Autodesk Inventor part; units mm, degrees
(part 2 of 2)
  arc A229 (57.1329, 113.815) -> (59.0329, 111.915) centre (59.0329, 113.815) ccw
  line L194 (78.8671, 123.4514) -> (78.8671, 113.815)
  arc A230 (78.8671, 123.4514) -> (76.9671, 125.3514) centre (76.9671, 123.4514) ccw
  line L195 (76.9671, 125.3514) -> (71.42, 125.3514)
  line L196 (71.42, 111.915) -> (76.9671, 111.915)
  arc A231 (76.9671, 111.915) -> (78.8671, 113.815) centre (76.9671, 113.815) ccw
  arc A232 (64.58, 125.3514) -> (71.42, 125.3514) centre (68, 128.8174) ccw
  arc A233 (71.42, 111.915) -> (64.58, 111.915) centre (68, 108.495) ccw
  line L197 (57.1329, 12.5486) -> (57.1329, 22.185)
  arc A234 (57.1329, 12.5486) -> (59.0329, 10.6486) centre (59.0329, 12.5486) ccw
  line L198 (59.0329, 10.6486) -> (64.58, 10.6486)
  line L199 (64.58, 24.085) -> (59.0329, 24.085)
  arc A235 (59.0329, 24.085) -> (57.1329, 22.185) centre (59.0329, 22.185) ccw
  line L200 (78.8671, 12.5486) -> (78.8671, 22.185)
  arc A236 (76.9671, 10.6486) -> (78.8671, 12.5486) centre (76.9671, 12.5486) ccw
  line L201 (76.9671, 10.6486) -> (71.42, 10.6486)
  line L202 (71.42, 24.085) -> (76.9671, 24.085)
  arc A237 (78.8671, 22.185) -> (76.9671, 24.085) centre (76.9671, 22.185) ccw
  arc A238 (71.42, 10.6486) -> (64.58, 10.6486) centre (68, 7.1826) ccw
  arc A239 (64.58, 24.085) -> (71.42, 24.085) centre (68, 27.505) ccw
  arc A240 (27.6448, 91.2527) -> (44.7476, 108.3555) centre (-2.445, 138.4453) ccw
  arc A241 (27.6448, 91.2527) -> (28.102, 89.6852) centre (28.102, 90.5356) ccw
  arc A242 (46.3151, 107.8983) -> (44.7476, 108.3555) centre (45.4647, 107.8983) ccw
  line L203 (40.2804, 87.1341) -> (22.5335, 87.1334)
  line L204 (44.1891, 89.6852) -> (28.102, 89.6852)
  line L205 (46.3151, 91.8112) -> (46.3151, 107.8983)
  arc A243 (44.1891, 89.6852) -> (46.3151, 91.8112) centre (44.1891, 91.8112) ccw
  arc A244 (27.1963, 78.4533) -> (28.6868, 78.3895) centre (28.007, 79.9485) ccw
  arc A245 (28.6868, 78.3895) -> (40.8045, 85.614) centre (6.3199, 129.6804) ccw
  line L206 (21.3459, 81.6253) -> (27.1963, 78.4533)
  line L207 (30.5408, 76.64) -> (37.2048, 73.0269)
  arc A246 (40.8045, 85.614) -> (40.2804, 87.1341) centre (40.2804, 86.2837) ccw
  arc A247 (91.2524, 108.3555) -> (108.3552, 91.2527) centre (138.445, 138.4453) ccw
  arc A248 (107.898, 89.6852) -> (108.3552, 91.2527) centre (107.898, 90.5356) ccw
  arc A249 (91.2524, 108.3555) -> (89.6849, 107.8983) centre (90.5353, 107.8983) ccw
  line L208 (91.8109, 89.6852) -> (107.898, 89.6852)
  line L209 (89.6849, 91.8112) -> (89.6849, 107.8983)
  arc A250 (89.6849, 91.8112) -> (91.8109, 89.6852) centre (91.8109, 91.8112) ccw
  arc A251 (108.3552, 44.7479) -> (91.2524, 27.6451) centre (138.445, -2.4447) ccw
  arc A252 (108.3552, 44.7479) -> (107.898, 46.3154) centre (107.898, 45.465) ccw
  arc A253 (89.6849, 28.1023) -> (91.2524, 27.6451) centre (90.5353, 28.1023) ccw
  line L210 (91.8109, 46.3154) -> (107.898, 46.3154)
  line L211 (89.6849, 44.1894) -> (89.6849, 28.1023)
  arc A254 (91.8109, 46.3154) -> (89.6849, 44.1894) centre (91.8109, 44.1894) ccw
  arc A255 (30.5752, 77.4043) -> (44.1261, 85.6969) centre (8.4389, 128.7951) ccw
  arc A256 (44.7901, 85.2067) -> (44.1261, 85.6969) centre (44.3973, 85.3694) ccw
  arc A257 (30.5752, 77.4043) -> (30.5408, 76.64) centre (30.7434, 77.0138) ccw
  line L212 (44.7901, 85.2067) -> (40.1822, 74.0823)
  arc A258 (37.2048, 73.0269) -> (40.1822, 74.0823) centre (38.2181, 74.8959) ccw
  line L213 (30.5408, 59.3606) -> (37.2048, 62.9737)
  arc A259 (40.1822, 61.9183) -> (37.2048, 62.9737) centre (38.2181, 61.1047) ccw
  arc A260 (44.1261, 50.3037) -> (30.5752, 58.5963) centre (8.4389, 7.2055) ccw
  arc A261 (44.1261, 50.3037) -> (44.7901, 50.7939) centre (44.3973, 50.6312) ccw
  arc A262 (30.5408, 59.3606) -> (30.5752, 58.5963) centre (30.7434, 58.9868) ccw
  line L214 (44.7901, 50.7939) -> (40.1822, 61.9183)
  line L215 (105.4592, 76.64) -> (98.7952, 73.0269)
  arc A263 (91.8739, 85.6969) -> (105.4248, 77.4043) centre (127.5611, 128.7951) ccw
  arc A264 (91.8739, 85.6969) -> (91.2099, 85.2067) centre (91.6027, 85.3694) ccw
  arc A265 (105.4592, 76.64) -> (105.4248, 77.4043) centre (105.2566, 77.0138) ccw
  line L216 (91.2099, 85.2067) -> (95.8178, 74.0823)
  arc A266 (95.8178, 74.0823) -> (98.7952, 73.0269) centre (97.7819, 74.8959) ccw
  line L217 (105.4592, 59.3606) -> (98.7952, 62.9737)
  arc A267 (98.7952, 62.9737) -> (95.8178, 61.9183) centre (97.7819, 61.1047) ccw
  arc A268 (105.4248, 58.5963) -> (91.8739, 50.3037) centre (127.5611, 7.2055) ccw
  arc A269 (91.2099, 50.7939) -> (91.8739, 50.3037) centre (91.6027, 50.6312) ccw
  arc A270 (105.4248, 58.5963) -> (105.4592, 59.3606) centre (105.2566, 58.9868) ccw
  line L218 (91.2099, 50.7939) -> (95.8178, 61.9183)
  line L219 (59.3603, 105.4595) -> (62.9734, 98.7955)
  arc A271 (61.918, 95.8181) -> (62.9734, 98.7955) centre (61.1044, 97.7822) ccw
  arc A272 (50.3034, 91.8742) -> (58.596, 105.4251) centre (7.2052, 127.5614) ccw
  arc A273 (50.3034, 91.8742) -> (50.7936, 91.2102) centre (50.6309, 91.603) ccw
  arc A274 (59.3603, 105.4595) -> (58.596, 105.4251) centre (58.9865, 105.2569) ccw
  line L220 (50.7936, 91.2102) -> (61.918, 95.8181)
  line L221 (76.6397, 105.4595) -> (73.0266, 98.7955)
  arc A275 (73.0266, 98.7955) -> (74.082, 95.8181) centre (74.8956, 97.7822) ccw
  arc A276 (77.404, 105.4251) -> (85.6966, 91.8742) centre (128.7948, 127.5614) ccw
  arc A277 (85.2064, 91.2102) -> (85.6966, 91.8742) centre (85.3691, 91.603) ccw
  arc A278 (77.404, 105.4251) -> (76.6397, 105.4595) centre (77.0135, 105.2569) ccw
  line L222 (85.2064, 91.2102) -> (74.082, 95.8181)
  line L223 (59.3603, 30.5411) -> (62.9734, 37.2051)
  arc A279 (62.9734, 37.2051) -> (61.918, 40.1825) centre (61.1044, 38.2184) ccw
  arc A280 (58.596, 30.5755) -> (50.3034, 44.1264) centre (7.2052, 8.4392) ccw
  arc A281 (50.7936, 44.7904) -> (50.3034, 44.1264) centre (50.6309, 44.3976) ccw
  arc A282 (58.596, 30.5755) -> (59.3603, 30.5411) centre (58.9865, 30.7437) ccw
  line L224 (50.7936, 44.7904) -> (61.918, 40.1825)
  line L225 (76.6397, 30.5411) -> (73.0266, 37.2051)
  arc A283 (85.6966, 44.1264) -> (77.404, 30.5755) centre (128.7948, 8.4392) ccw
  arc A284 (85.6966, 44.1264) -> (85.2064, 44.7904) centre (85.3691, 44.3976) ccw
  arc A285 (76.6397, 30.5411) -> (77.404, 30.5755) centre (77.0135, 30.7437) ccw
  line L226 (85.2064, 44.7904) -> (74.082, 40.1825)
  arc A286 (74.082, 40.1825) -> (73.0266, 37.2051) centre (74.8956, 38.2184) ccw
  circle A287 centre (68, 68) radius 24.5933
  arc A288 (44.7476, 27.6451) -> (27.6448, 44.7479) centre (-2.445, -2.4447) ccw
  arc A289 (44.7476, 27.6451) -> (46.3151, 28.1023) centre (45.4647, 28.1023) ccw
  arc A290 (28.102, 46.3154) -> (27.6448, 44.7479) centre (28.102, 45.465) ccw
  line L227 (46.3151, 44.1894) -> (46.3151, 28.1023)
  line L228 (44.1891, 46.3154) -> (28.102, 46.3154)
  arc A291 (46.3151, 44.1894) -> (44.1891, 46.3154) centre (44.1891, 44.1894) ccw
  line L229 (64.2924, 102.9057) -> (67.1209, 97.6888)
  arc A292 (67.1209, 97.6888) -> (68.8791, 97.6888) centre (68, 98.1654) ccw
  line L230 (71.7076, 102.9057) -> (68.8791, 97.6888)
  arc A293 (65.6558, 104.2572) -> (70.3442, 104.2572) centre (68, 108.4916) ccw
  arc A294 (65.6558, 104.2572) -> (64.2924, 102.9057) centre (65.1715, 103.3823) ccw
  arc A295 (71.7076, 102.9057) -> (70.3442, 104.2572) centre (70.8285, 103.3823) ccw
  line L231 (64.2924, 33.0943) -> (67.1209, 38.3112)
  arc A296 (68.8791, 38.3112) -> (67.1209, 38.3112) centre (68, 37.8346) ccw
  line L232 (71.7076, 33.0943) -> (68.8791, 38.3112)
  arc A297 (70.3442, 31.7428) -> (65.6558, 31.7428) centre (68, 27.5084) ccw
  arc A298 (64.2924, 33.0943) -> (65.6558, 31.7428) centre (65.1715, 32.6177) ccw
  arc A299 (70.3442, 31.7428) -> (71.7076, 33.0943) centre (70.8285, 32.6177) ccw
  line L233 (33.0946, 71.7079) -> (38.3115, 68.8794)
  arc A300 (38.3115, 67.1212) -> (38.3115, 68.8794) centre (37.8349, 68.0003) ccw
  line L234 (33.0946, 64.2927) -> (38.3115, 67.1212)
  arc A301 (31.7431, 65.6561) -> (31.7431, 70.3445) centre (27.5087, 68.0003) ccw
  arc A302 (33.0946, 71.7079) -> (31.7431, 70.3445) centre (32.618, 70.8288) ccw
  arc A303 (31.7431, 65.6561) -> (33.0946, 64.2927) centre (32.618, 65.1718) ccw
  line L235 (102.906, 71.7079) -> (97.6891, 68.8794)
  arc A304 (97.6891, 68.8794) -> (97.6891, 67.1212) centre (98.1657, 68.0003) ccw
  line L236 (102.906, 64.2927) -> (97.6891, 67.1212)
  arc A305 (104.2575, 70.3445) -> (104.2575, 65.6561) centre (108.4919, 68.0003) ccw
  arc A306 (104.2575, 70.3445) -> (102.906, 71.7079) centre (103.3826, 70.8288) ccw
  arc A307 (102.906, 64.2927) -> (104.2575, 65.6561) centre (103.3826, 65.1718) ccw
  circle A308 centre (7.7484, 68) radius 1.6
  circle A309 centre (128.2516, 68) radius 1.6
  circle A310 centre (68, 128.2516) radius 1.6
  circle A311 centre (68, 7.7484) radius 1.6
  arc A312 (4.7048, 71.2684) -> (4.7048, 64.7316) centre (8.3141, 68) ccw
  arc A313 (5.9986, 61.3754) -> (4.7048, 64.7316) centre (0.9986, 61.3754) ccw
  arc A314 (4.7048, 71.2684) -> (5.9986, 74.6246) centre (0.9986, 74.6246) ccw
  arc A315 (131.2952, 64.7316) -> (131.2952, 71.2684) centre (127.6859, 68) ccw
  arc A316 (131.2952, 64.7316) -> (130.0014, 61.3754) centre (135.0014, 61.3754) ccw
  arc A317 (130.0014, 74.6246) -> (131.2952, 71.2684) centre (135.0014, 74.6246) ccw
  arc A318 (71.2684, 131.2952) -> (64.7316, 131.2952) centre (68, 127.6859) ccw
  arc A319 (71.2684, 131.2952) -> (74.6246, 130.0014) centre (74.6246, 135.0014) ccw
  arc A320 (61.3754, 130.0014) -> (64.7316, 131.2952) centre (61.3754, 135.0014) ccw
  arc A321 (64.7316, 4.7048) -> (71.2684, 4.7048) centre (68, 8.3141) ccw
  arc A322 (64.7316, 4.7048) -> (61.3754, 5.9986) centre (61.3754, 0.9986) ccw
  arc A323 (74.6246, 5.9986) -> (71.2684, 4.7048) centre (74.6246, 0.9986) ccw
  line L237 (17, 83.6623) -> (17, 82.8671)
  arc A324 (18.2965, 85.5345) -> (21.7007, 86.9517) centre (-0.1983, 134.7566) ccw
  arc A325 (18.2965, 85.5345) -> (17, 83.6623) centre (19, 83.6623) ccw
  arc A326 (22.5335, 87.1334) -> (21.7007, 86.9517) centre (22.5336, 85.1334) ccw
  line L238 (18, 81.8671) -> (20.3926, 81.8671)
  arc A327 (17, 82.8671) -> (18, 81.8671) centre (18, 82.8671) ccw
  arc A328 (21.3459, 81.6253) -> (20.3926, 81.8671) centre (20.3926, 79.8671) ccw
  line L239 (40.2804, 48.8659) -> (22.5335, 48.8666)
  arc A329 (28.6868, 57.6105) -> (27.1963, 57.5467) centre (28.007, 56.0515) ccw
  arc A330 (40.8045, 50.386) -> (28.6868, 57.6105) centre (6.3199, 6.3196) ccw
  line L240 (21.3459, 54.3747) -> (27.1963, 57.5467)
  arc A331 (40.2804, 48.8659) -> (40.8045, 50.386) centre (40.2804, 49.7163) ccw
  line L241 (17, 52.3377) -> (17, 53.1329)
  arc A332 (21.7007, 49.0483) -> (18.2965, 50.4655) centre (-0.1983, 1.2434) ccw
  arc A333 (17, 52.3377) -> (18.2965, 50.4655) centre (19, 52.3377) ccw
  arc A334 (21.7007, 49.0483) -> (22.5335, 48.8666) centre (22.5336, 50.8666) ccw
  line L242 (18, 54.1329) -> (20.3926, 54.1329)
  arc A335 (18, 54.1329) -> (17, 53.1329) centre (18, 53.1329) ccw
  arc A336 (20.3926, 54.1329) -> (21.3459, 54.3747) centre (20.3926, 56.1329) ccw
  line L243 (95.7196, 87.1341) -> (113.4665, 87.1334)
  arc A337 (107.3132, 78.3895) -> (108.8037, 78.4533) centre (107.993, 79.9485) ccw
  arc A338 (95.1955, 85.614) -> (107.3132, 78.3895) centre (129.6801, 129.6804) ccw
  line L244 (114.6541, 81.6253) -> (108.8037, 78.4533)
  arc A339 (95.7196, 87.1341) -> (95.1955, 85.614) centre (95.7196, 86.2837) ccw
  line L245 (119, 83.6623) -> (119, 82.8671)
  arc A340 (114.2993, 86.9517) -> (117.7035, 85.5345) centre (136.1983, 134.7566) ccw
  arc A341 (119, 83.6623) -> (117.7035, 85.5345) centre (117, 83.6623) ccw
  arc A342 (114.2993, 86.9517) -> (113.4665, 87.1334) centre (113.4664, 85.1334) ccw
  line L246 (118, 81.8671) -> (115.6074, 81.8671)
  arc A343 (118, 81.8671) -> (119, 82.8671) centre (118, 82.8671) ccw
  arc A344 (115.6074, 81.8671) -> (114.6541, 81.6253) centre (115.6074, 79.8671) ccw
  line L247 (95.7196, 48.8659) -> (113.4665, 48.8666)
  arc A345 (108.8037, 57.5467) -> (107.3132, 57.6105) centre (107.993, 56.0515) ccw
  arc A346 (107.3132, 57.6105) -> (95.1955, 50.386) centre (129.6801, 6.3196) ccw
  line L248 (114.6541, 54.3747) -> (108.8037, 57.5467)
  arc A347 (95.1955, 50.386) -> (95.7196, 48.8659) centre (95.7196, 49.7163) ccw
  line L249 (119, 52.3377) -> (119, 53.1329)
  arc A348 (117.7035, 50.4655) -> (114.2993, 49.0483) centre (136.1983, 1.2434) ccw
  arc A349 (117.7035, 50.4655) -> (119, 52.3377) centre (117, 52.3377) ccw
  arc A350 (113.4665, 48.8666) -> (114.2993, 49.0483) centre (113.4664, 50.8666) ccw
  line L250 (118, 54.1329) -> (115.6074, 54.1329)
  arc A351 (119, 53.1329) -> (118, 54.1329) centre (118, 53.1329) ccw
  arc A352 (114.6541, 54.3747) -> (115.6074, 54.1329) centre (115.6074, 56.1329) ccw
  line L251 (48.8662, 40.2807) -> (48.8669, 22.5339)
  arc A353 (57.547, 27.1966) -> (57.6108, 28.6871) centre (56.0518, 28.0073) ccw
  arc A354 (57.6108, 28.6871) -> (50.3863, 40.8048) centre (6.3199, 6.3202) ccw
  line L252 (54.375, 21.3462) -> (57.547, 27.1966)
  arc A355 (50.3863, 40.8048) -> (48.8662, 40.2807) centre (49.7166, 40.2807) ccw
  line L253 (52.338, 17.0003) -> (53.1332, 17.0003)
  arc A356 (50.4658, 18.2968) -> (49.0486, 21.701) centre (1.2437, -0.198) ccw
  arc A357 (50.4658, 18.2968) -> (52.338, 17.0003) centre (52.338, 19.0003) ccw
  arc A358 (48.8669, 22.5339) -> (49.0486, 21.701) centre (50.8669, 22.5339) ccw
  line L254 (54.1332, 18.0003) -> (54.1332, 20.3929)
  arc A359 (53.1332, 17.0003) -> (54.1332, 18.0003) centre (53.1332, 18.0003) ccw
  arc A360 (54.375, 21.3462) -> (54.1332, 20.3929) centre (56.1332, 20.3929) ccw
  line L255 (87.1344, 40.2807) -> (87.1337, 22.5339)
  arc A361 (78.3898, 28.6871) -> (78.4536, 27.1966) centre (79.9488, 28.0073) ccw
  arc A362 (85.6143, 40.8048) -> (78.3898, 28.6871) centre (129.6807, 6.3202) ccw
  line L256 (81.6256, 21.3462) -> (78.4536, 27.1966)
  arc A363 (87.1344, 40.2807) -> (85.6143, 40.8048) centre (86.284, 40.2807) ccw
  line L257 (83.6626, 17.0003) -> (82.8674, 17.0003)
  arc A364 (86.952, 21.701) -> (85.5348, 18.2968) centre (134.7569, -0.198) ccw
  arc A365 (83.6626, 17.0003) -> (85.5348, 18.2968) centre (83.6626, 19.0003) ccw
  line L258 (87.1344, 95.7199) -> (87.1337, 113.4668)
  arc A366 (86.952, 21.701) -> (87.1337, 22.5339) centre (85.1337, 22.5339) ccw
  line L259 (81.8674, 18.0003) -> (81.8674, 20.3929)
  arc A367 (81.8674, 18.0003) -> (82.8674, 17.0003) centre (82.8674, 18.0003) ccw
  arc A368 (81.8674, 20.3929) -> (81.6256, 21.3462) centre (79.8674, 20.3929) ccw
  line L260 (48.8662, 95.7199) -> (48.8669, 113.4668)
  arc A369 (57.6108, 107.3135) -> (57.547, 108.804) centre (56.0518, 107.9933) ccw
  arc A370 (50.3863, 95.1958) -> (57.6108, 107.3135) centre (6.3199, 129.6804) ccw
  line L261 (54.375, 114.6544) -> (57.547, 108.804)
  arc A371 (48.8662, 95.7199) -> (50.3863, 95.1958) centre (49.7166, 95.7199) ccw
  line L262 (52.338, 119.0003) -> (53.1332, 119.0003)
  arc A372 (49.0486, 114.2996) -> (50.4658, 117.7038) centre (1.2437, 136.1986) ccw
  arc A373 (52.338, 119.0003) -> (50.4658, 117.7038) centre (52.338, 117.0003) ccw
  arc A374 (49.0486, 114.2996) -> (48.8669, 113.4668) centre (50.8669, 113.4667) ccw
  line L263 (54.1332, 118.0003) -> (54.1332, 115.6077)
  arc A375 (54.1332, 118.0003) -> (53.1332, 119.0003) centre (53.1332, 118.0003) ccw
  arc A376 (54.1332, 115.6077) -> (54.375, 114.6544) centre (56.1332, 115.6077) ccw
  arc A377 (78.4536, 108.804) -> (78.3898, 107.3135) centre (79.9488, 107.9933) ccw
  arc A378 (85.6143, 95.1958) -> (87.1344, 95.7199) centre (86.284, 95.7199) ccw
  arc A379 (78.3898, 107.3135) -> (85.6143, 95.1958) centre (129.6807, 129.6804) ccw
  line L264 (81.6256, 114.6544) -> (78.4536, 108.804)
  line L265 (83.6626, 119.0003) -> (82.8674, 119.0003)
  arc A380 (85.5348, 117.7038) -> (86.952, 114.2996) centre (134.7569, 136.1986) ccw
  arc A381 (85.5348, 117.7038) -> (83.6626, 119.0003) centre (83.6626, 117.0003) ccw
  arc A382 (87.1337, 113.4668) -> (86.952, 114.2996) centre (85.1337, 113.4667) ccw
  line L266 (81.8674, 118.0003) -> (81.8674, 115.6077)
  arc A383 (82.8674, 119.0003) -> (81.8674, 118.0003) centre (82.8674, 118.0003) ccw
  arc A384 (81.6256, 114.6544) -> (81.8674, 115.6077) centre (79.8674, 115.6077) ccw
  line L267 (0, 83.4142) -> (0, 84.8722)
  arc A385 (0, 83.4142) -> (0.2929, 82.7071) centre (1, 83.4142) ccw
  line L268 (4.5341, 78.4659) -> (0.2929, 82.7071)
  line L269 (5.9986, 61.0697) -> (5.9986, 61.3754)
  line L270 (0, 52.5858) -> (0, 51.1198)
  line L271 (4.5341, 57.5341) -> (0.2929, 53.2929)
  arc A386 (4.5341, 57.5341) -> (5.9986, 61.0697) centre (0.9986, 61.0697) ccw
  arc A387 (0.2929, 53.2929) -> (0, 52.5858) centre (1, 52.5858) ccw
  line L272 (61.0697, 5.9986) -> (61.3754, 5.9986)
  line L273 (52.5858, 0) -> (51.1278, 0)
  line L274 (57.5341, 4.5341) -> (53.2929, 0.2929)
  arc A388 (61.0697, 5.9986) -> (57.5341, 4.5341) centre (61.0697, 0.9986) ccw
  arc A389 (52.5858, 0) -> (53.2929, 0.2929) centre (52.5858, 1) ccw
  line L275 (74.9303, 5.9986) -> (74.6246, 5.9986)
  arc A390 (78.4659, 4.5341) -> (74.9303, 5.9986) centre (74.9303, 0.9986) ccw
  line L276 (83.4142, 0) -> (84.8801, 0)
  arc A391 (82.7071, 0.2929) -> (83.4142, 0) centre (83.4142, 1) ccw
  line L277 (78.4659, 4.5341) -> (82.7071, 0.2929)
  line L278 (130.0014, 61.0697) -> (130.0014, 61.3754)
  line L279 (136, 52.5858) -> (136, 51.1278)
  arc A392 (136, 52.5858) -> (135.7071, 53.2929) centre (135, 52.5858) ccw
  line L280 (131.4659, 57.5341) -> (135.7071, 53.2929)
  arc A393 (130.0014, 61.0697) -> (131.4659, 57.5341) centre (135.0014, 61.0697) ccw
  line L281 (130.0014, 74.9303) -> (130.0014, 74.6246)
  arc A394 (131.4659, 78.4659) -> (130.0014, 74.9303) centre (135.0014, 74.9303) ccw
  line L282 (136, 83.4142) -> (136, 84.8802)
  arc A395 (135.7071, 82.7071) -> (136, 83.4142) centre (135, 83.4142) ccw
  line L283 (131.4659, 78.4659) -> (135.7071, 82.7071)
  line L284 (74.9303, 130.0014) -> (74.6246, 130.0014)
  line L285 (83.4142, 136) -> (84.8722, 136)
  arc A396 (83.4142, 136) -> (82.7071, 135.7071) centre (83.4142, 135) ccw
  line L286 (78.4659, 131.4659) -> (82.7071, 135.7071)
  arc A397 (74.9303, 130.0014) -> (78.4659, 131.4659) centre (74.9303, 135.0014) ccw
  line L287 (61.0697, 130.0014) -> (61.3754, 130.0014)
  arc A398 (57.5341, 131.4659) -> (61.0697, 130.0014) centre (61.0697, 135.0014) ccw
  line L288 (52.5858, 136) -> (51.1198, 136)
  arc A399 (53.2929, 135.7071) -> (52.5858, 136) centre (52.5858, 135) ccw
  line L289 (57.5341, 131.4659) -> (53.2929, 135.7071)
  point P0 (0, 0)
  constraints: 380 point on circle, 292 end point, 199 centre point, 130 tangent, 58 horizontal, 38 vertical, 18 parallel, 11 perpendicular, 5 coincident, 3 collinear, 454 other
extrude "Extrusion1" add sketch "Sketch1" along normal blind 2 contours A25 A11 L32 A12 L33 A31 L39 A30 A27 A28 L38 A29 L34 A13 L35 A14 A26 A15 L37 A16 L43 A32 L40 A33 A36 A35 L41 A34 L42 A18 L36 A17 A23 A19 L44 A20 L46 A38 L45 A39 A40 A111 L91 A37 L115 A144 L114 A143 A24 A21 L47 A22 L49 A42 L50 A41 A43 A142 L112 A141 L113 A10 L48 A9
body "Solid1"
